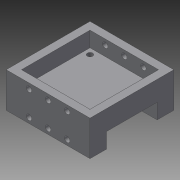
# Autodesk Inventor part: Lead_Screw_Motor_Mount
Saved by Autodesk Inventor 2015 (Build 190159000, 159)
## iProperties
Created: 2014-12-28
Part Number: Lead_Screw_Motor_Mount
Material: Generic
Document SubType Name: Modeling
Designer: Drew
Density: 1 g/cm^3
Appearance: Default
Author: Drew
Autodesk Inventor part; units mm, degrees
ref_plane "YZ Plane" through (0, 0, 0) normal (1, 0, 0) x (0, 1, 0)
ref_plane "XZ Plane" through (0, 0, 0) normal (0, 1, 0) x (-1, 0, 0)
ref_plane "XY Plane" through (0, 0, 0) normal (0, 0, 1) x (1, 0, 0)
sketch "Sketch1" plane through (0, 0, 0) normal (0, 1, 0) x (-1, 0, 0)
  line L0 (-34.85, -34.85) -> (34.85, -34.85)
  line L1 (34.85, -34.85) -> (34.85, 34.85)
  line L2 (34.85, 34.85) -> (-34.85, 34.85)
  line L3 (-34.85, 34.85) -> (-34.85, -34.85)
  line L4 (-34.85, -34.85) -> (34.85, 34.85) construction
  line L5 (34.85, -34.85) -> (-34.85, 34.85) construction
  line L6 (-28.5, -28.5) -> (28.5, -28.5)
  line L7 (28.5, -28.5) -> (28.5, 28.5)
  line L8 (28.5, 28.5) -> (-28.5, 28.5)
  line L9 (-28.5, 28.5) -> (-28.5, -28.5)
  line L10 (-28.5, -28.5) -> (28.5, 28.5) construction
  line L11 (28.5, -28.5) -> (-28.5, 28.5) construction
  point P0 (0, 0)
  dimension "d6" = 57
  dimension "d7" = 57
  dimension "d8" = 6.35
  constraints: 24 end point, 4 midpoint, 4 parallel, 2 horizontal, 2 perpendicular, 1 point on line
  measures "d6" distance between parallel lines of L8 L6
  measures "d7" distance between parallel lines of L9 L7
  measures "d8" distance between parallel lines of L1 L7
extrude "Extrusion1" add sketch "Sketch1" along normal blind 12.7
sketch "Sketch2" plane through (0, 0, 0) normal (0, -1, 0) x (1, 0, 0)
  line L0 (-34.85, -34.85) -> (34.85, -34.85)
  line L1 (34.85, -34.85) -> (34.85, 34.85)
  line L2 (34.85, 34.85) -> (-34.85, 34.85)
  line L3 (-34.85, 34.85) -> (-34.85, -34.85)
  line L4 (-34.85, -34.85) -> (34.85, 34.85) construction
  line L5 (34.85, -34.85) -> (-34.85, 34.85) construction
  point P0 (0, 0)
  point P1 (34.85, -34.85)
  constraints: 12 end point, 2 midpoint, 2 parallel, 2 point on line, 1 horizontal, 1 perpendicular
extrude "Extrusion2" add sketch "Sketch2" along normal blind 3.81
sketch "Sketch3" plane through (0, -3.81, 0) normal (0, -1, 0) x (1, 0, 0)
  line L0 (34.85, 34.85) -> (34.85, -34.85) projected
  line L1 (-34.85, 34.85) -> (34.85, 34.85)
  line L2 (34.85, 34.85) -> (34.85, 21)
  line L3 (34.85, 21) -> (-34.85, 21)
  line L4 (-34.85, 21) -> (-34.85, 34.85)
  line L5 (-43.7088, 0) -> (41.6447, 0)
  line L6 (-34.85, -34.85) -> (34.85, -34.85)
  line L7 (34.85, -34.85) -> (34.85, -21)
  line L8 (34.85, -21) -> (-34.85, -21)
  line L9 (-34.85, -21) -> (-34.85, -34.85)
  dimension "d10" = 42
  constraints: 18 end point, 5 symmetric about line, 2 horizontal, 2 parallel, 1 perpendicular, 1 point on line
  measures "d10" distance between parallel lines of L8 L3
extrude "Extrusion3" add sketch "Sketch3" along normal blind 12.7
sketch "Sketch4" plane through (-34.85, 12.7, 34.85) normal (0, 0, 1) x (1, 0, 0)
  line L0 (-8.0078, -24.765) -> (75.1101, -24.765)
  circle A0 centre (18.975, -24.765) radius 2.25
  circle A1 centre (34.85, -24.765) radius 2.25
  line L1 (34.85, 4.0697) -> (34.85, -35.8474)
  line L2 (0, -29.21) -> (0, 0) projected
  line L3 (0, -14.605) -> (69.7, -14.605)
  line L4 (69.7, -29.21) -> (69.7, 0) projected
  circle A2 centre (50.725, -24.765) radius 2.25
  circle A3 centre (18.975, -4.445) radius 2.25
  circle A4 centre (34.85, -4.445) radius 2.25
  circle A5 centre (50.725, -4.445) radius 2.25
  point P0 (34.85, -12.7)
  dimension "d38" = 4.5
  dimension "d39" = 4.5
  dimension "d41" = 31.75
  dimension "d42" = 10.16
  constraints: 6 centre point, 6 end point, 4 point on line, 4 symmetric about line, 2 midpoint, 1 horizontal, 1 vertical, 4 other
  measures "d38" diameter of A0
  measures "d39" diameter of A1
  measures "d41" diameter of A0.centre L1
  measures "d42" distance between parallel lines of L0 L3
extrude "Extrusion4" cut sketch "Sketch4" against normal through all contours A0 L0 | L0 A0 | A1 L1 L0 | L0 L1 A1 | A1 L0 L1 | L0 A1 L1 | A2 L0 | L0 A2 | A4 L1 | L1 A4 | A3 | A5
sketch "Sketch5" plane through (0, 0, 0) normal (0, 1, 0) x (1, 0, 0)
  line L0 (0, -37.456) -> (0, 33.7968)
  line L1 (-33.5936, 0) -> (36.338, 0)
  circle A0 centre (23.57, -23.57) radius 2.25
  circle A1 centre (-23.57, -23.57) radius 2.25
  circle A2 centre (23.57, 23.57) radius 2.25
  circle A3 centre (-23.57, 23.57) radius 2.25
  point P0 (0, 0)
  dimension "d45" = 4.5
  dimension "d46" = 47.14
  dimension "d47" = 47.14
  constraints: 4 centre point, 4 end point, 3 symmetric about line, 2 point on line, 1 horizontal, 1 vertical, 3 other
  measures "d45" diameter of A0
  measures "d46" diameter of A0.centre L0
  measures "d47" diameter of A0.centre L1
extrude "Extrusion5" cut sketch "Sketch5" against normal blind 12.7
equation "\"d7\" = d6"
equation "\"d39\" = d38"
equation "\"d47\" = d46"
body "Solid1"
